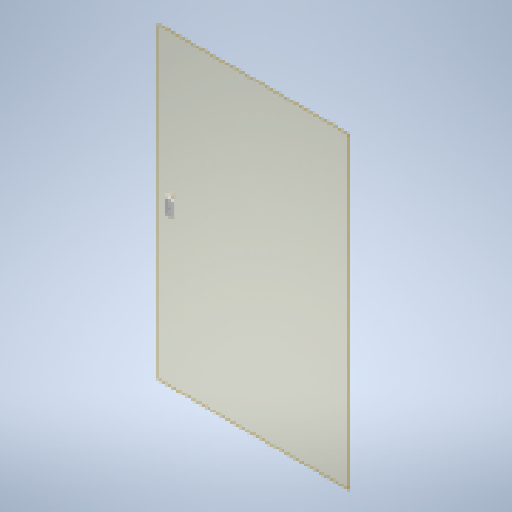
# Autodesk Inventor part: Union abajo
Saved by Autodesk Inventor 2023 (Build 270158000, 158)
## iProperties
Created: 2023-05-14
Part Number: Union abajo
Material: Genérico
Document SubType Name: Modeling
Designer: sergi
Density: 1 g/cm^3
Appearance: Valor por defecto
Author: sergi
Autodesk Inventor part; units mm, degrees
ref_plane "YZ Plane" through (0, 0, 0) normal (1, 0, 0) x (0, 1, 0)
ref_plane "XZ Plane" through (0, 0, 0) normal (0, 1, 0) x (-1, 0, 0)
ref_plane "XY Plane" through (0, 0, 0) normal (0, 0, 1) x (1, 0, 0)
ref_plane "Plano de trabajo1" through (0, 0, 0) normal (0, 0, 1) x (1, 0, 0)
sketch "Boceto1" plane through (0, 0, 0) normal (0, 0, 1) x (1, 0, 0)
  circle A0 centre (108.375, -226.9) radius 1.5
  circle A1 centre (108.375, -327.280446) radius 1.5
  line L0 (58.475, -218.4) -> (58.475, -213.4)
  line L1 (58.475, -213.4) -> (80.675, -213.4)
  line L2 (80.675, -213.4) -> (80.675, -218.4)
  line L3 (58.475, -218.4) -> (80.675, -218.4)
  line L4 (99.475, -248.4) -> (104.475, -248.4)
  line L5 (104.475, -248.4) -> (104.475, -268.4)
  line L6 (104.475, -268.4) -> (99.475, -268.4)
  line L7 (99.475, -330.5) -> (99.475, -268.4)
  line L8 (99.475, -330.5) -> (44.375, -330.5)
  line L9 (44.375, -330.5) -> (44.375, -223.4)
  line L10 (99.475, -223.4) -> (44.375, -223.4)
  line L11 (99.475, -248.4) -> (99.475, -223.4)
  line L12 (98.375, -209.4) -> (88.675, -209.4)
  line L13 (88.675, -209.4) -> (88.675, -176)
  line L14 (88.675, -176) -> (197.375, -176)
  line L15 (197.375, -176) -> (197.375, -326)
  line L16 (197.375, -326) -> (112.375, -326)
  line L17 (112.375, -326) -> (112.375, -223.4)
  arc A2 (112.375, -223.4) -> (98.375, -209.4) centre (98.375, -223.4) ccw
  line L18 (29.999359, -209.4) -> (29.999359, -326)
  line L19 (29.999359, -326) -> (20.625, -326)
  line L20 (20.625, -326) -> (20.625, -288)
  line L21 (20.625, -288) -> (9.375, -288)
  line L22 (9.375, -288) -> (9.375, -176)
  line L23 (9.375, -176) -> (20.625, -176)
  line L24 (20.625, -176) -> (20.625, -209.4)
  line L25 (20.625, -209.4) -> (29.999359, -209.4)
  circle A3 centre (69.375, -196) radius 1.6
  circle A4 centre (44.375, -196) radius 1.6
  circle A5 centre (215.275, -317.3) radius 1.5
  circle A6 centre (2.725, -309.3) radius 1.5
  circle A7 centre (2.725, -317.7) radius 1.5
  circle A8 centre (215.275, -311.6) radius 1.5
  line L26 (212.375, -161) -> (-5.625, -161)
  line L27 (-5.625, -161) -> (-5.625, -303)
  line L28 (-5.625, -303) -> (5.625, -303)
  line L29 (5.625, -303) -> (5.625, -306)
  line L30 (5.625, -306) -> (-1.875, -306)
  line L31 (-1.875, -306) -> (-1.875, -321)
  line L32 (-1.875, -321) -> (5.625, -321)
  line L33 (5.625, -321) -> (5.625, -341)
  line L34 (5.625, -341) -> (212.375, -341)
  line L35 (212.375, -341) -> (212.375, -321)
  line L36 (212.375, -321) -> (218.675, -321)
  line L37 (218.675, -321) -> (218.675, -307.9)
  line L38 (218.675, -307.9) -> (212.375, -307.9)
  line L39 (212.375, -307.9) -> (212.375, -161)
  circle A9 centre (143.025, -170) radius 1.5
  circle A10 centre (94.675, -170) radius 1.5
  circle A11 centre (191.375, -170) radius 1.5
  circle A12 centre (33.999359, -226.9) radius 1.5
  circle A13 centre (33.999359, -327.540446) radius 1.5
  circle A14 centre (143.025, -152) radius 1.5
  circle A15 centre (94.675, -152) radius 1.5
  circle A16 centre (191.375, -152) radius 1.5
  line L40 (-5.625, -161) -> (212.375, -161)
  line L41 (212.375, -161) -> (212.375, -14.1)
  line L42 (212.375, -14.1) -> (218.675, -14.1)
  line L43 (218.675, -14.1) -> (218.675, -1)
  line L44 (218.675, -1) -> (212.375, -1)
  line L45 (212.375, -1) -> (212.375, 19)
  line L46 (212.375, 19) -> (5.625, 19)
  line L47 (5.625, 19) -> (5.625, -1)
  line L48 (5.625, -1) -> (-1.875, -1)
  line L49 (-1.875, -1) -> (-1.875, -16)
  line L50 (-1.875, -16) -> (5.625, -16)
  line L51 (5.625, -16) -> (5.625, -19)
  line L52 (5.625, -19) -> (-5.625, -19)
  line L53 (-5.625, -19) -> (-5.625, -161)
  circle A17 centre (215.275, -4.7) radius 1.5
  circle A18 centre (2.725, -12.7) radius 1.5
  circle A19 centre (2.725, -4.3) radius 1.5
  circle A20 centre (215.275, -10.4) radius 1.5
  line L54 (91.875, 14.8) -> (91.875, -3.3)
  line L55 (91.875, -3.3) -> (83.875, -3.3)
  line L56 (83.875, -3.3) -> (83.875, 14.8)
  line L57 (83.875, 14.8) -> (91.875, 14.8)
  line L58 (163.175, 8.8) -> (163.175, 2.3)
  line L59 (163.175, 2.3) -> (156.675, 2.3)
  line L60 (156.675, 2.3) -> (156.675, 8.8)
  line L61 (156.675, 8.8) -> (163.175, 8.8)
  line L62 (145.075, 8.8) -> (145.075, 2.3)
  line L63 (145.075, 2.3) -> (138.575, 2.3)
  line L64 (138.575, 2.3) -> (138.575, 8.8)
  line L65 (138.575, 8.8) -> (145.075, 8.8)
  line L66 (102.375, 2.3) -> (102.375, 8.8)
  line L67 (102.375, 8.8) -> (108.875, 8.8)
  line L68 (108.875, 8.8) -> (108.875, 2.3)
  line L69 (108.875, 2.3) -> (102.375, 2.3)
  line L70 (184.675, 8.8) -> (184.675, 2.3)
  line L71 (184.675, 2.3) -> (178.175, 2.3)
  line L72 (178.175, 2.3) -> (178.175, 8.8)
  line L73 (178.175, 8.8) -> (184.675, 8.8)
  line L74 (126.975, 8.8) -> (126.975, 2.3)
  line L75 (126.975, 2.3) -> (120.475, 2.3)
  line L76 (120.475, 2.3) -> (120.475, 8.8)
  line L77 (120.475, 8.8) -> (126.975, 8.8)
  circle A21 centre (44.375, -126) radius 1.6
  circle A22 centre (69.375, -126) radius 1.6
  line L78 (20.625, -146) -> (9.375, -146)
  line L79 (9.375, -146) -> (9.375, -34)
  line L80 (9.375, -34) -> (20.625, -34)
  line L81 (20.625, -34) -> (20.625, 4)
  line L82 (20.625, 4) -> (49.475, 4)
  line L83 (49.475, 4) -> (49.475, -112.6)
  line L84 (49.475, -112.6) -> (20.625, -112.6)
  line L85 (20.625, -112.6) -> (20.625, -146)
  line L86 (88.675, -146) -> (88.675, -10.3)
  line L87 (88.675, -10.3) -> (197.375, -10.3)
  line L88 (197.375, -10.3) -> (197.375, -146)
  line L89 (197.375, -146) -> (88.675, -146)
  line L90 (220.675, 19) -> (220.675, -161)
  line L91 (-7.625, 19) -> (-7.625, -161)
  line L92 (212.875, -14.6) -> (212.875, -161)
  line L93 (-6.125, -161) -> (-6.125, -18.5)
  line L94 (-7.625, -161) -> (2.375, -161)
  line L95 (2.375, -161) -> (2.375, -171)
  line L96 (2.375, -171) -> (-9.625, -171)
  line L97 (-9.625, -171) -> (-9.625, -151)
  line L98 (-9.625, -151) -> (2.375, -151)
  line L99 (2.375, -151) -> (2.375, -171)
  line L100 (2.375, -151) -> (-1.625, -151)
  line L101 (-1.625, -151) -> (-1.625, -171)
  line L102 (2.375, -151) -> (2.375, -156)
  line L103 (2.375, -156) -> (-1.625, -156)
  line L104 (2.375, -171) -> (2.375, -166)
  line L105 (2.375, -166) -> (-1.625, -166)
  circle A23 centre (-1.625, -156) radius 1
  circle A24 centre (-1.625, -166) radius 1
  line L106 (-7.625, -161) -> (-6.125, -161)
  line L107 (-6.125, -18.5) -> (5.125, -18.5)
  line L108 (5.125, -18.5) -> (5.125, -16.5)
  line L109 (5.125, -16.5) -> (-2.375, -16.5)
  line L110 (-2.375, -16.5) -> (-2.375, -0.5)
  line L111 (-2.375, -0.5) -> (5.125, -0.5)
  line L112 (5.125, -0.5) -> (5.125, 19.5)
  line L113 (5.125, 19.5) -> (212.875, 19.5)
  line L114 (212.875, 19.5) -> (212.875, -0.5)
  line L115 (212.875, -0.5) -> (219.175, -0.5)
  line L116 (219.175, -0.5) -> (219.175, -14.6)
  line L117 (219.175, -14.6) -> (212.875, -14.6)
  line L118 (212.875, -161) -> (220.675, -161)
  arc A25 (220.675, 19) -> (218.675, 21) centre (218.675, 19) ccw
  line L119 (218.675, 21) -> (-5.625, 21)
  arc A26 (-5.625, 21) -> (-7.625, 19) centre (-5.625, 19) ccw
  circle A27 centre (216.675, -156) radius 1.5
  point P0 (0, 0)
  dimension "d0" = 10
  dimension "d1" = 10
  dimension "d2" = 12
  dimension "d3" = 20
  dimension "d4" = 4
  dimension "d5" = 5
  dimension "d6" = 5
  dimension "d7" = 2
  dimension "d8" = 2
  constraints: 25 end point, 7 point on line, 5 perpendicular, 2 centre point, 2 coincident, 2 parallel, 1 horizontal
  measures "d0" distance of L91.end L94.end
  measures "d1" distance of L94.end L95.end
  measures "d2" distance of L97.end L98.end
  measures "d3" distance of L96.end L97.end
  measures "d4" distance of L98.end L100.end
  measures "d5" distance of L98.end L102.end
  measures "d6" distance of L95.end L104.end
  measures "d7" diameter of A23
  measures "d8" diameter of A24
extrude "Extrusión1" add sketch "Boceto1" along normal blind 3 contours L95 L105 A24 L101 L26 | L26 L101 A23 L103 L99 | L101 A24 L96 L27 L26 | L26 L53 L98 L101 A23 | L95 L96 L101 A24 L105 | L103 A23 L101 L98 L99 | L94 L93 L98 L53 | L27 L96 L97 L98 L91 L94 | L94 L91 L98 L93
sketch "Boceto2" plane through (0, 0, 0) normal (0, 0, -1) x (-1, 0, 0)
  line L0 (7.625, 19) -> (7.625, -161)
  line L1 (-2.375, -151) -> (9.625, -151)
  line L2 (-2.375, -171) -> (-2.375, -151)
  line L3 (9.625, -171) -> (-2.375, -171)
  line L4 (9.625, -151) -> (9.625, -171)
  circle A0 centre (1.625, -166) radius 1
  circle A1 centre (1.625, -156) radius 1
  line L5 (-14.191374, -161) -> (6.008626, -161)
  line L6 (7.625, 19) -> (7.625, -161)
  arc A2 (7.625, 19) -> (5.625, 21) centre (5.625, 19) ccw
  line L7 (5.625, 21) -> (-218.675, 21)
  arc A3 (-218.675, 21) -> (-220.675, 19) centre (-218.675, 19) ccw
  line L8 (-220.675, 19) -> (-220.675, -161)
  line L9 (-222.291374, -161) -> (-209.991374, -161)
  line L10 (-208.375, -161) -> (-208.375, 9.8)
  line L11 (-208.375, 9.8) -> (-12.575, 9.8)
  line L12 (-12.575, 9.8) -> (-12.575, -161)
  circle A4 centre (-215.275, -4.7) radius 1.2
  circle A5 centre (-2.725, -4.3) radius 1.2
  circle A6 centre (-2.725, -12.7) radius 1.2
  circle A7 centre (-215.275, -10.4) radius 1.2
  line L13 (6.008626, -161) -> (-14.191374, -161)
  line L14 (-14.191374, -161) -> (-14.191374, -337)
  line L15 (-14.191374, -337) -> (-209.991374, -337)
  line L16 (-209.991374, -337) -> (-209.991374, -161)
  line L17 (-209.991374, -161) -> (-222.291374, -161)
  line L18 (-222.291374, -161) -> (-222.291374, -346.2)
  arc A8 (-222.291374, -346.2) -> (-220.291374, -348.2) centre (-220.291374, -346.2) ccw
  line L19 (4.008626, -348.2) -> (-220.291374, -348.2)
  arc A9 (4.008626, -348.2) -> (6.008626, -346.2) centre (4.008626, -346.2) ccw
  line L20 (6.008626, -161) -> (6.008626, -346.2)
  circle A10 centre (-216.891374, -311.6) radius 1.2
  circle A11 centre (-4.341374, -309.3) radius 1.2
  circle A12 centre (-4.341374, -317.7) radius 1.2
  circle A13 centre (-216.891374, -317.3) radius 1.2
  line L21 (-2.375, -151) -> (9.625, -151)
  line L22 (9.625, -151) -> (9.625, -171)
  line L23 (9.625, -171) -> (-2.375, -171)
  line L24 (-2.375, -171) -> (-2.375, -151)
  circle A14 centre (1.625, -166) radius 1
  circle A15 centre (1.625, -156) radius 1
  point P0 (0, 0)
  point P1 (6.098425, -151)
  point P2 (7.625, -171)
  point P3 (6.008626, -171)
  constraints: 1 other
sketch "Boceto2 outline for Extrusión2" plane through (0, 0, 0) normal (0, 0, -1) x (-1, 0, 0)
  line L0 (6.008626, -161) -> (6.008626, -171)
  line L1 (6.098425, -151) -> (6.008626, -161)
  line L2 (9.625, -151) -> (6.098425, -151)
  line L3 (9.625, -171) -> (9.625, -151)
  line L4 (6.008626, -171) -> (9.625, -171)
extrude "Extrusión2" add sketch "Boceto2 outline for Extrusión2" along normal blind 8
fillet "Empalme1" radius 2 1 edges at (-9.625, -161, 3)
sketch "Boceto4" plane through (-9.625, -171, -8) normal (-1, 0, 0) x (0, 0, 1)
  line L0 (9, 20) -> (9, 0) projected
  line L1 (0, 20) -> (9, 20) projected
  line L2 (0, 0) -> (0, 20) projected
  line L3 (0, 0) -> (9, 0) projected
  line L4 (4.1, 262) -> (4.1, -242)
  line L5 (4.1, 20) -> (4.1, 15)
  circle A0 centre (4.1, 15) radius 1
  line L6 (8, 0) -> (0, 0) projected
  line L7 (4.1, 0) -> (4.1, 5)
  circle A1 centre (4.1, 5) radius 1
  point P0 (8, 171)
  dimension "d14" = 5
  dimension "d15" = 2
  dimension "d16" = 5
  dimension "d17" = 2
  constraints: 6 end point, 6 point on line, 2 centre point, 2 coincident, 1 vertical, 2 other
  measures "d14" distance of L5.start L5.end
  measures "d15" diameter of A0
  measures "d16" distance of L7.start L7.end
  measures "d17" diameter of A1
hole "Agujero1" at (-9.625, -166, -3.9) at (-9.625, -156, -3.9) direction (1, 0, 0) diameter 2.4 end through all
fillet "Empalme2" radius 2 4 edges at (-7.8617, -151, -8) (-7.8168, -171, -8) (2.375, -151, 1.5) (2.375, -171, 1.5)
